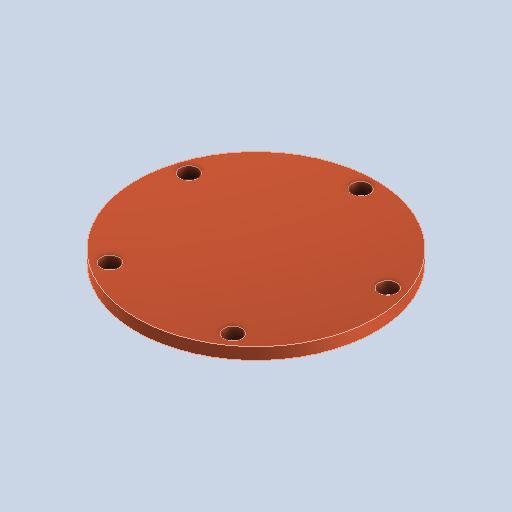
# Autodesk Inventor part: 35
Saved by Autodesk Inventor 2025.1 (Build 291241000, 241)
## iProperties
Created: 2024-09-17
Part Number: 35
Material: Copper, Alloy
Document SubType Name: Modeling
Designer: ffogue
Density: 8.92 g/cm^3
Appearance: Copper - Satin
Author: ffogue
Autodesk Inventor part; units mm, degrees
ref_plane "YZ Plane" through (0, 0, 0) normal (1, 0, 0) x (0, 1, 0)
ref_plane "XZ Plane" through (0, 0, 0) normal (0, 1, 0) x (-1, 0, 0)
ref_plane "XY Plane" through (0, 0, 0) normal (0, 0, 1) x (1, 0, 0)
sketch "Sketch1" plane through (0, 0, 0) normal (0, 0, 1) x (1, 0, 0)
  circle A0 centre (0, 0) radius 20
  dimension "d0" = 40
  constraints: 1 centre point, 1 coincident
  measures "d0" diameter of A0
extrude "Extrusion1" add sketch "Sketch1" along normal blind 2
sketch "Sketch2" plane through (0, 0, 2) normal (0, 0, 1) x (1, 0, 0)
  circle A0 centre (0, 0) radius 17.5 construction
  point P0 (0, 17.5)
  dimension "d3" = 35
  constraints: 2 vertical alignment, 1 coincident, 2 other
hole "Hole1" at (0, 17.5, 2) direction (0, 0, -1) diameter 3 depth 2
pattern_circular "Circular Pattern1" count 5 over 360 about axis through (0, 0, 0) along (0, 0, 1) of "Hole1"
body "Solid1"
